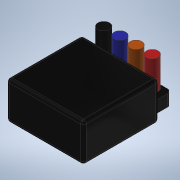
# Autodesk Inventor part: MC402CR
Saved by Autodesk Inventor 2020.2 (Build 242310000, 310)
## iProperties
Created: 2013-08-04
Part Number: MC402CR
Material: ABS Plastic
Document SubType Name: Modeling
Designer: Kentaro2
Density: 3.1152 g/cm^3
Mass: 30 g
Surface Area: 33.5905 cm^2
Volume: 9.6302 cm^3
Appearance: 光沢 - 黒
Author: Kentaro2
Autodesk Inventor part; units mm, degrees
ref_plane "YZ Plane" through (0, 0, 0) normal (1, 0, 0) x (0, 1, 0)
ref_plane "XZ Plane" through (0, 0, 0) normal (0, 1, 0) x (-1, 0, 0)
sketch "スケッチ1" plane through (0, 0, 0) normal (0, 0, 1) x (1, 0, 0)
  line L0 (0, 0) -> (26.2, 0)
  line L1 (26.2, 0) -> (26.2, -25.7)
  line L2 (26.2, -25.7) -> (0, -25.7)
  line L3 (0, -25.7) -> (0, 0)
  dimension "d0" = 25.7
  dimension "d1" = 26.2
  constraints: 8 end point, 2 perpendicular, 1 horizontal, 1 vertical
  measures "d0" distance of L0.end L1.end
  measures "d1" distance of L1.end L2.end
extrude "外形" add sketch "スケッチ1" along normal blind 12.9
ref_plane "作業平面1" through (0, 0, 6.45) normal (0, 0, 1) x (1, 0, 0)
sketch "スケッチ2" plane through (0, 0, 6.45) normal (0, 0, 1) x (1, 0, 0)
  line L0 (0, 0) -> (26.2, 0) projected
  line L1 (0, 0) -> (26.2, 0) projected
  line L2 (0.6, 0) -> (0.6, 5)
  line L3 (0.6, 5) -> (25.6, 5)
  line L4 (25.6, 5) -> (25.6, 0)
  line L5 (13.1, 0) -> (13.1, 3.4882)
  dimension "d5" = 5
  dimension "d6" = 25
  constraints: 8 end point, 3 perpendicular, 2 point on line, 1 midpoint, 1 parallel, 1 other
  measures "d5" distance between parallel lines of L0 L3
  measures "d6" distance between parallel lines of L4 L2
extrude "突起部" add sketch "スケッチ2" against normal blind 4
chamfer "面取り1" distance 1 angle 45 2 edges at (0.6, 5, 4.45) (25.6, 5, 4.45)
fillet "フィレット1" radius 1 12 edges at (0, 0, 6.45) (0, -25.7, 6.45) (26.2, -25.7, 6.45) (13.1, -25.7, 12.9) (26.2, -12.85, 12.9) (26.2, -12.85, 0) (0, -12.85, 12.9) (13.1, 0, 12.9) (13.1, 0, 0) (13.1, -25.7, 0) (26.2, 0, 6.45) (0, -12.85, 0)
fillet "フィレット2" radius 1 4 edges at (25.6, 4, 4.45) (24.6, 5, 4.45) (1.6, 5, 4.45) (0.6, 4, 4.45)
sketch "スケッチ3" plane through (0, 0, 6.45) normal (0, 0, 1) x (1, 0, 0)
  arc A0 (2.0142, 5) -> (1.3071, 4.7071) centre (2.0142, 4) ccw projected
  line L0 (0.6, 4) -> (1.3071, 4.7071) projected
  line L1 (0.6, 4) -> (0.6, -0.0835) projected
  arc A1 (1, 0) -> (0.6, -0.0835) centre (1, -1) ccw projected
  line L2 (25.2, 0) -> (1, 0) projected
  arc A2 (25.6, -0.0835) -> (25.2, 0) centre (25.2, -1) ccw projected
  line L3 (25.6, -0.0835) -> (25.6, 3.5858) projected
  arc A3 (25.6, 3.5858) -> (25.3071, 4.2929) centre (24.6, 3.5858) ccw projected
  line L4 (24.8929, 4.7071) -> (25.3071, 4.2929) projected
  arc A4 (24.8929, 4.7071) -> (24.1858, 5) centre (24.1858, 4) ccw projected
  line L5 (24.1858, 5) -> (2.0142, 5) projected
  line L6 (4.85, 2.5808) -> (21.35, 2.5808)
  line L7 (13.1, 5) -> (13.1, 0.3828)
  point P0 (0, 0)
  point P1 (10.35, 2.5808)
  point P2 (15.85, 2.5808)
  dimension "d14" = 5.5
  dimension "d15" = 16.5
  constraints: 4 end point, 2 perpendicular, 2 point on line, 2 symmetric about line, 1 midpoint
  measures "d14" distance of point (15.85, 2.581) point (10.35, 2.581)
  measures "d15" distance of L6.start L6.end
sketch "スケッチ4" plane through (0, 0, 6.45) normal (0, 0, 1) x (1, 0, 0)
  circle A0 centre (4.85, 2.5808) radius 2
  circle A1 centre (10.35, 2.5808) radius 2
  circle A2 centre (15.85, 2.5808) radius 2
  circle A3 centre (21.35, 2.5808) radius 2
  point P0 (0, 0)
  dimension "d16" = 4
  dimension "d17" = 4
  dimension "d18" = 4
  dimension "d19" = 4
  constraints: 4 centre point, 4 coincident
  measures "d16" diameter of A0
  measures "d17" diameter of A1
  measures "d18" diameter of A2
  measures "d19" diameter of A3
extrude "押し出し3" add sketch "スケッチ4" along normal blind 10
equation "\"d14\" = 0.333333 * d15"
